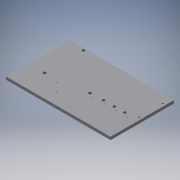
# Autodesk Inventor part: board_15x15x0.5
Saved by Autodesk Inventor 2017 (Build 210142000, 142)
## iProperties
Created: 2019-02-04
Part Number: board_15x15x0.5
Material: Generic
Document SubType Name: Modeling
Designer: S346559073
Density: 1 g/cm^3
Appearance: Default
Author: S346559073
Autodesk Inventor part; units mm, degrees
ref_plane "YZ Plane" through (0, 0, 0) normal (1, 0, 0) x (0, 1, 0)
ref_plane "XZ Plane" through (0, 0, 0) normal (0, 1, 0) x (-1, 0, 0)
ref_plane "XY Plane" through (0, 0, 0) normal (0, 0, 1) x (1, 0, 0)
sketch "Sketch1" plane through (0, 0, 0) normal (0, 1, 0) x (-1, 0, 0)
  line L0 (0, 0) -> (435.102, 0)
  line L1 (435.102, 0) -> (435.102, -279.4)
  line L2 (435.102, -279.4) -> (0, -279.4)
  line L3 (0, -279.4) -> (0, 0)
  dimension "d0" = 435.102
  dimension "d1" = 279.4
  constraints: 8 end point, 2 parallel, 1 horizontal, 1 perpendicular
  measures "d0" distance of L1.end L2.end
  measures "d1" distance of L0.end L1.end
extrude "Extrusion1" add sketch "Sketch1" along normal blind 12.7
sketch "Sketch2" plane through (0, 12.7, 0) normal (0, 1, 0) x (1, 0, 0)
  line L0 (0, 0) -> (0, 279.4) projected
  line L1 (-435.102, 279.4) -> (-435.102, 0) projected
  line L2 (-435.102, 0) -> (0, 0) projected
  line L3 (-190.5, 139.7) -> (0, 139.7)
  line L4 (0, 279.4) -> (-435.102, 279.4) projected
  line L5 (0, 279.4) -> (0, 139.7)
  line L6 (0, 0) -> (0, 139.7)
  circle A0 centre (-11.5062, 138.303) radius 2.667
  circle A1 centre (-11.5062, 242.697) radius 2.667
  dimension "d8" = 5.334
  dimension "d10" = 5.334
  dimension "d20" = 11.5062
  dimension "d21" = 11.5062
  constraints: 6 end point, 2 centre point, 1 collinear, 1 midpoint, 1 perpendicular
  measures "d8" diameter of A0
  measures "d10" diameter of A1
  measures "d20" distance from line of A1.centre L0
  measures "d21" distance from line of L0 A0.centre
extrude "Extrusion2" cut sketch "Sketch2" against normal blind 12.7 contours A0 L3 | L3 A0 | A1
thread "Thread1" size "12-24 UNC" class "2B" standard "ANSI Unified Screw Threads" full length
thread "Thread2" size "12-24 UNC" class "2B" standard "ANSI Unified Screw Threads" full length
sketch "Sketch9" plane through (0, 12.7, 0) normal (0, 1, 0) x (1, 0, 0)
  line L0 (-435.102, 279.4) -> (-435.102, 0) projected
  line L1 (0, 279.4) -> (-435.102, 279.4) projected
  line L2 (-228.6, 279.4) -> (-114.6048, 279.4)
  circle A0 centre (-228.6, 165.4048) radius 1.905
  circle A1 centre (-276.352, 165.4048) radius 1.905
  point P0 (0, 0)
  dimension "d59" = 3.81
  dimension "d61" = 113.9952
  dimension "d63" = 3.81
  dimension "d64" = 47.752
  constraints: 2 centre point, 2 end point, 2 point on line
  measures "d59" diameter of A0
  measures "d61" distance from line of L1 A0.centre
  measures "d63" diameter of A1
  measures "d64" distance of A1.centre A0.centre
extrude "Extrusion6" cut sketch "Sketch9" against normal blind 25.4
sketch "Sketch10" plane through (0, 12.7, 0) normal (0, 1, 0) x (1, 0, 0)
  circle A0 centre (-73.9111, 98.5347) radius 1.9812 projected
  line L0 (-73.9111, 98.5347) -> (-179.5995, 98.5347)
  circle A1 centre (-179.5995, 98.5347) radius 1.905
  point P0 (0, 0)
  dimension "d67" = 3.81
  constraints: 2 end point, 1 centre point, 1 coincident, 1 horizontal
  measures "d67" diameter of A1
sketch "Sketch11" plane through (0, 12.7, 0) normal (0, 1, 0) x (1, 0, 0)
  circle A0 centre (-138.6966, 96.5535) radius 1.9812 projected
  circle A1 centre (-138.6966, 96.5535) radius 1.9812
  circle A2 centre (-73.9111, 98.5347) radius 1.9812 projected
  circle A3 centre (-73.9111, 98.5347) radius 1.9812
  circle A4 centre (-138.6966, 96.5535) radius 1.9812 projected
  circle A5 centre (-189.4966, 96.5535) radius 1.905
  circle A6 centre (-138.6966, 274.9457) radius 1.905
  circle A7 centre (-189.4966, 276.8507) radius 1.905
  line L0 (-233.5122, 296.5851) -> (-202.1873, 265.2602)
  line L1 (-198.1568, 261.2297) -> (-195.5777, 258.6506)
  line L2 (-147.3568, 261.2297) -> (-144.7777, 258.6506)
  line L3 (-182.7122, 296.5851) -> (-151.3873, 265.2602)
  line L4 (-147.3154, 108.6372) -> (-144.7363, 111.2163)
  line L5 (-151.3873, 104.6481) -> (-182.7122, 73.3232)
  line L6 (-195.5777, 111.2577) -> (-198.1568, 108.6786)
  line L7 (-202.1873, 104.6481) -> (-233.5122, 73.3232)
  circle A8 centre (-228.6, 165.4048) radius 1.905 projected
  circle A9 centre (-276.352, 165.4048) radius 1.905 projected
  circle A10 centre (-11.5062, 138.303) radius 2.667 projected
  circle A11 centre (-11.5062, 242.697) radius 2.667 projected
  line L8 (-435.102, 0) -> (0, 0) projected
  line L9 (0, 0) -> (0, 279.4) projected
  line L10 (0, 279.4) -> (-435.102, 279.4) projected
  line L11 (-435.102, 279.4) -> (-435.102, 0) projected
  line L12 (-189.2001, 247.8995) -> (-37.7952, 247.8995)
  line L13 (-189.2001, 133.1005) -> (-39.5732, 133.1005)
  line L14 (-138.6966, 133.1005) -> (-138.6966, 122.2293)
  line L15 (-195.5777, 122.2293) -> (-196.8672, 259.9401)
  line L16 (-144.7777, 258.6506) -> (-147.3147, 111.2577)
  line L17 (-147.3147, 111.2577) -> (-195.5777, 111.2577)
  line L18 (-195.5777, 111.2577) -> (-195.5777, 122.2293)
  line L19 (-138.6966, 122.2293) -> (-195.5777, 122.2293)
  line L20 (-138.6966, 122.2293) -> (-138.6966, 111.1549)
  circle A12 centre (-138.6966, 111.1549) radius 1.905
  circle A13 centre (-189.2001, 111.2577) radius 1.905
  circle A14 centre (-138.6966, 96.5535) radius 1.9812
  circle A15 centre (-189.4966, 96.5535) radius 1.905
  circle A16 centre (-111.9102, 274.9457) radius 1.9812
  circle A17 centre (-138.6966, 274.9457) radius 1.905
  circle A18 centre (-189.4966, 276.8507) radius 1.905
  circle A19 centre (-228.6, 165.4048) radius 1.905 projected
  circle A20 centre (-228.6, 165.4048) radius 1.905
  circle A21 centre (-276.352, 165.4048) radius 1.905 projected
  circle A22 centre (-276.352, 165.4048) radius 1.905
  dimension "d72" = 3.81
  dimension "d77" = 3.81
  dimension "d78" = 3.81
  dimension "d127" = 21.8842
  dimension "d128" = 10.8712
  dimension "d129" = 11.0744
  dimension "d130" = 3.81
  dimension "d131" = 3.81
  constraints: 34 end point, 14 centre point, 8 coincident, 3 concentric, 3 point on line, 2 horizontal, 2 perpendicular, 1 midpoint, 1 vertical, 28 other
  measures "d72" diameter of A5
  measures "d77" diameter of A6
  measures "d78" diameter of A7
  measures "d127" distance from line of L4.end L13
  measures "d128" distance of L14.start L14.end
  measures "d129" distance of L14.end L20.end
  measures "d130" diameter of A12
  measures "d131" diameter of A13
extrude "Extrusion7" add sketch "Sketch10" against normal blind 12.7 contours A0
extrude "Extrusion8" cut sketch "Sketch11" against normal blind 12.7 contours A5
sketch "Sketch12" plane through (0, 12.7, 0) normal (0, 1, 0) x (1, 0, 0)
  circle A0 centre (-111.9102, 274.9457) radius 1.9812 projected
  circle A1 centre (-111.9102, 274.9457) radius 1.9812
  circle A2 centre (-50.2837, 276.9269) radius 1.9812 projected
  circle A3 centre (-50.2837, 276.9269) radius 1.9812
  point P0 (0, 0)
  constraints: 2 centre point, 2 coincident, 1 concentric
extrude "Extrusion9" add sketch "Sketch12" against normal blind 12.7
sketch "Sketch13" plane through (0, 12.7, 0) normal (0, 1, 0) x (1, 0, 0)
  circle A0 centre (-189.4966, 96.5535) radius 1.905 projected
  circle A1 centre (-138.6966, 96.5535) radius 1.9812 projected
  line L0 (-435.102, 279.4) -> (0, 279.4) projected
  circle A2 centre (-138.6966, 273.3548) radius 1.905
  circle A3 centre (-189.4966, 273.3548) radius 1.905
  point P0 (0, 0)
  dimension "d79" = 3.81
  dimension "d80" = 3.81
  constraints: 2 centre point
  measures "d79" diameter of A2
  measures "d80" diameter of A3
extrude "Extrusion10" cut sketch "Sketch13" against normal blind 12.7 contours A2 | A3
sketch "Sketch15" plane through (0, 0, 0) normal (0, -1, 0) x (1, 0, 0)
  circle A0 centre (-189.4966, -273.3548) radius 1.905 projected
  circle A1 centre (-189.4966, -273.3548) radius 1.905
  circle A2 centre (-138.6966, -273.3548) radius 1.905 projected
  circle A3 centre (-138.6966, -273.3548) radius 1.905
  point P0 (0, 0)
  constraints: 2 centre point, 2 coincident
extrude "Extrusion12" add sketch "Sketch15" against normal blind 12.7
sketch "Sketch16" plane through (0, 12.7, 0) normal (0, 1, 0) x (1, 0, 0)
  circle A0 centre (-301.5668, 273.3548) radius 1.905
  circle A1 centre (-253.8148, 273.3548) radius 1.905
  point P0 (0, 0)
  dimension "d89" = 3.81
  dimension "d90" = 3.81
  dimension "d91" = 47.752
  constraints: 2 centre point
  measures "d89" diameter of A0
  measures "d90" diameter of A1
  measures "d91" distance of A0.centre A1.centre
extrude "Extrusion13" cut sketch "Sketch16" against normal blind 12.7
sketch "Sketch17" plane through (0, 12.7, 0) normal (0, 1, 0) x (1, 0, 0)
  circle A0 centre (-228.6, 165.4048) radius 1.905 projected
  circle A1 centre (-228.6, 165.4048) radius 1.905
  circle A2 centre (-276.352, 165.4048) radius 1.905 projected
  circle A3 centre (-276.352, 165.4048) radius 1.905
  point P0 (0, 0)
  constraints: 2 centre point, 2 coincident
extrude "Extrusion14" add sketch "Sketch17" against normal blind 12.7
sketch "Sketch18" plane through (0, 12.7, 0) normal (0, 1, 0) x (1, 0, 0)
  circle A0 centre (-154.6206, 259.3143) radius 6.35
  circle A1 centre (-199.1169, 258.3518) radius 6.35
  circle A2 centre (-211.7706, 121.6705) radius 6.35
  circle A3 centre (-148.3169, 155.711) radius 6.35
  circle A4 centre (-363.982, 103.99) radius 6.35
  circle A5 centre (-363.982, 266.5172) radius 6.35
  line L0 (-435.102, 279.4) -> (-435.102, 0) projected
  line L1 (-182.8964, 164.601) -> (-33.2695, 164.601) projected
  line L2 (-192.48, 267.7748) -> (-192.48, 273.9984) projected
  point P0 (0, 0)
  dimension "d102" = 12.7
  dimension "d103" = 12.7
  dimension "d105" = 12.7
  dimension "d106" = 12.7
  dimension "d107" = 12.7
  dimension "d109" = 12.7
  dimension "d110" = 71.12
  dimension "d111" = 71.12
  dimension "d124" = 8.89
  dimension "d126" = 6.6369
  constraints: 6 centre point
  measures "d102" diameter of A0
  measures "d103" diameter of A1
  measures "d105" diameter of A2
  measures "d106" diameter of A3
  measures "d107" diameter of A4
  measures "d109" diameter of A5
  measures "d110" distance from line of A4.centre L0
  measures "d111" distance from line of L0 A5.centre
  measures "d124" distance from line of L1 A3.centre
  measures "d126" distance from line of L2 A1.centre
extrude "Extrusion15" cut sketch "Sketch18" against normal blind 12.7 contours A0 | A1 | A2 | A3
sketch "Sketch19" plane through (0, 12.7, 0) normal (0, 1, 0) x (1, 0, 0)
  circle A0 centre (-363.982, 270.4356) radius 6.35
  line L0 (-435.102, 279.4) -> (-435.102, 0) projected
  circle A1 centre (-363.982, 99.0328) radius 6.35
  circle A2 centre (-148.3169, 155.711) radius 6.35 projected
  line L1 (-182.8964, 164.601) -> (-33.2695, 164.601) projected
  point P0 (0, 0)
  dimension "d114" = 12.7
  dimension "d116" = 71.12
  dimension "d117" = 12.7
  dimension "d119" = 71.12
  constraints: 2 centre point
  measures "d114" diameter of A0
  measures "d116" distance from line of L0 A0.centre
  measures "d117" diameter of A1
  measures "d119" distance from line of L0 A1.centre
extrude "Extrusion16" cut sketch "Sketch19" against normal blind 12.7 contours A0 | A1
sketch "Sketch21" plane through (0, 12.7, 0) normal (0, 1, 0) x (1, 0, 0)
  circle A0 centre (-138.6966, 96.5535) radius 1.9812
  circle A1 centre (-138.6966, 96.5535) radius 1.9812
  circle A2 centre (-73.9111, 98.5347) radius 1.9812
  circle A3 centre (-73.9111, 98.5347) radius 1.9812
  circle A4 centre (-138.6966, 96.5535) radius 1.9812
  circle A5 centre (-189.4966, 96.5535) radius 1.905
  circle A6 centre (-138.6966, 274.9457) radius 1.905
  circle A7 centre (-189.4966, 276.8507) radius 1.905
  line L0 (-198.1568, 261.2297) -> (-195.5777, 258.6506)
  line L1 (-147.3568, 261.2297) -> (-144.7777, 258.6506)
  line L2 (-147.3154, 108.6372) -> (-144.7363, 111.2163)
  line L3 (-151.3873, 104.6481) -> (-182.7122, 73.3232)
  line L4 (-195.5777, 111.2577) -> (-198.1568, 108.6786)
  line L5 (-202.1873, 104.6481) -> (-233.5122, 73.3232)
  circle A8 centre (-228.6, 273.3548) radius 1.905
  circle A9 centre (-276.352, 273.3548) radius 1.905
  circle A10 centre (-111.9102, 274.9457) radius 1.9812
  circle A11 centre (-138.6966, 96.5535) radius 1.9812
  circle A12 centre (-50.2837, 276.9269) radius 1.9812
  circle A13 centre (-11.5062, 138.303) radius 2.667
  circle A14 centre (-11.5062, 242.697) radius 2.667
  line L6 (-189.2001, 247.8995) -> (-37.7952, 247.8995)
  line L7 (-189.2001, 133.1005) -> (-39.5732, 133.1005)
  line L8 (-138.6966, 133.1005) -> (-138.6966, 122.2293)
  line L9 (-195.5777, 122.2293) -> (-196.8672, 259.9401)
  line L10 (-144.7777, 258.6506) -> (-147.3147, 111.2577)
  line L11 (-147.3147, 111.2577) -> (-195.5777, 111.2577)
  line L12 (-195.5777, 111.2577) -> (-195.5777, 122.2293)
  line L13 (-138.6966, 122.2293) -> (-195.5777, 122.2293)
  line L14 (-138.6966, 122.2293) -> (-138.6966, 111.1549)
  circle A15 centre (-138.6966, 111.1549) radius 1.905
  circle A16 centre (-189.2001, 111.2577) radius 1.905
  point P0 (0, 0)
  point P1 (-202.1873, 265.2602)
  point P2 (-151.3873, 265.2602)
  dimension "d132" = 3.81
  dimension "d133" = 3.81
  dimension "d134" = 3.81
  dimension "d135" = 21.8842
  dimension "d136" = 10.8712
  dimension "d137" = 11.0744
  dimension "d138" = 3.81
  dimension "d139" = 3.81
  constraints: 30 end point, 17 centre point, 3 coincident, 3 point on line, 2 horizontal, 2 perpendicular, 1 midpoint, 1 vertical, 24 other
  measures "d132" diameter of A5
  measures "d133" diameter of A6
  measures "d134" diameter of A7
  measures "d135" distance from line of L2.end L7
  measures "d136" distance of L8.start L8.end
  measures "d137" distance of L8.end L14.end
  measures "d138" diameter of A15
  measures "d139" diameter of A16
extrude "Extrusion17" cut sketch "Sketch21" against normal blind 12.7 contours A15 | A16 L11 | L11 A16
sketch "Sketch22" plane through (0, 12.7, 0) normal (0, 1, 0) x (1, 0, 0)
  circle A0 centre (-138.6966, 289.5514) radius 1.905 projected
  circle A1 centre (-138.6966, 289.5514) radius 1.905
  circle A2 centre (-189.4966, 291.4564) radius 1.905 projected
  circle A3 centre (-189.4966, 291.4564) radius 1.905
  circle A4 centre (-253.8148, 273.3548) radius 1.905 projected
  circle A5 centre (-253.8148, 273.3548) radius 1.905
  circle A6 centre (-301.5668, 273.3548) radius 1.905 projected
  circle A7 centre (-301.5668, 273.3548) radius 1.905
  circle A8 centre (-189.4966, 96.5535) radius 1.905 projected
  circle A9 centre (-189.4966, 96.5535) radius 1.905
  circle A10 centre (-138.6966, 96.5535) radius 1.9812 projected
  circle A11 centre (-138.6966, 96.5535) radius 1.9812
  point P0 (0, 0)
  constraints: 6 centre point, 6 coincident
extrude "Extrusion18" add sketch "Sketch22" against normal blind 12.7
sketch "Sketch24" plane through (-189.4966, 12.7, -291.4564) normal (0, 1, 0) x (1, 0, 0)
  circle A0 centre (50.8, -1.905) radius 1.905 projected
  circle A1 centre (50.8, -1.905) radius 1.905
  circle A2 centre (0, 0) radius 1.905 projected
  circle A3 centre (0, 0) radius 1.905
  point P0 (189.4966, -291.4564)
  constraints: 2 centre point, 2 coincident
extrude "Extrusion19" cut sketch "Sketch24" against normal blind 12.7
sketch "Sketch25" plane through (0, 12.7, 0) normal (0, 1, 0) x (1, 0, 0)
  circle A0 centre (-325.2254, 87.7397) radius 1.905
  circle A1 centre (-291.4597, 53.974) radius 1.905
  line L0 (-325.2254, 87.7397) -> (-291.4597, 53.974)
  point P0 (0, 0)
  dimension "d147" = 3.81
  dimension "d148" = 3.81
  dimension "d152" = 47.752
  constraints: 2 centre point, 2 end point, 1 coincident
  measures "d147" diameter of A0
  measures "d148" diameter of A1
  measures "d152" distance of L0.start L0.end
extrude "Extrusion20" cut sketch "Sketch25" against normal blind 12.7
sketch "Sketch26" plane through (0, 12.7, 0) normal (0, 1, 0) x (1, 0, 0)
  circle A0 centre (-88.2014, 111.1549) radius 1.905
  circle A1 centre (-138.6966, 111.1549) radius 1.905 projected
  circle A2 centre (-37.7062, 111.1549) radius 1.905
  point P0 (0, 0)
  dimension "d155" = 3.81
  dimension "d156" = 50.4952
  dimension "d157" = 3.81
  dimension "d158" = 50.4952
  constraints: 2 centre point
  measures "d155" diameter of A0
  measures "d156" distance of A0.centre A1.centre
  measures "d157" diameter of A2
  measures "d158" distance of A0.centre A2.centre
extrude "Extrusion21" cut sketch "Sketch26" against normal blind 12.7 contours A0 | A2
sketch "Sketch27" plane through (0, 12.7, 0) normal (0, 1, 0) x (1, 0, 0)
  circle A0 centre (-106.8659, 124.2105) radius 6.35
  circle A1 centre (-148.3169, 155.711) radius 6.35 projected
  circle A2 centre (-61.1072, 124.2105) radius 6.35
  point P0 (0, 0)
  dimension "d162" = 12.7
  dimension "d163" = 12.7
  constraints: 2 centre point
  measures "d162" diameter of A0
  measures "d163" diameter of A2
extrude "Extrusion22" cut sketch "Sketch27" against normal blind 12.7 contours A0 | A2
sketch "Sketch29" plane through (0, 12.7, 0) normal (0, 1, 0) x (1, 0, 0)
  circle A0 centre (-199.1169, 258.3518) radius 6.35 projected
  circle A1 centre (-199.1169, 258.3518) radius 6.35
  circle A2 centre (-154.6206, 259.3143) radius 6.35 projected
  circle A3 centre (-154.6206, 259.3143) radius 6.35
  point P0 (0, 0)
  constraints: 2 centre point, 2 coincident
extrude "Extrusion23" add sketch "Sketch29" against normal blind 12.7
body "Solid1"
